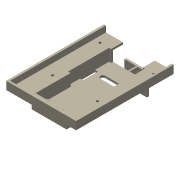
# Autodesk Inventor part: stat_plate
Saved by Autodesk Inventor 2022 (Build 260148000, 148)
## iProperties
Shininess: 64.0
Length Units: 11272
Angle Units: 11279
Time Units: 11290
Mass Units: 11286
Length Display Precision: 3
Angle Display Precision: 2
Created: 2002-04-25
Part Number: stat_plate
Document SubType Name: Modeling
Designer: Administrator
Density: 1 g/cm^3
Material: Generic
Appearance: Light Beige
Density: 0.0
Volumn: 0.0
Area: 0.0
PropertySet Name: Model Information
Control State: 0
Master: False
Checked Out: False
Author: Administrator
Autodesk Inventor part; units mm, degrees
ref_plane "YZ Plane" through (0, 0, 0) normal (1, 0, 0) x (0, 1, 0)
ref_plane "XZ Plane" through (0, 0, 0) normal (0, 1, 0) x (-1, 0, 0)
sketch "Sketch1" plane through (0, 0, 0) normal (0, 0, 1) x (1, 0, 0)
  line L0 (-52.4488, 14.7313) -> (-52.4488, 4.5713)
  line L1 (-52.4488, 4.5713) -> (36.4512, 4.5713)
  line L2 (36.4512, 4.5713) -> (36.4512, 14.7313)
  line L3 (36.4512, 14.7313) -> (-52.4488, 14.7313)
  dimension "d0" = 10.16
  dimension "d13" = 88.9
  constraints: 8 end point, 2 perpendicular, 1 horizontal, 1 parallel, 1 vertical
  measures "d0" distance of L0.start L0.end
  measures "d13" distance of L0.end L1.end
extrude "Extrusion1" add sketch "Sketch1" along normal blind 121.92
sketch "Sketch2" plane through (0, 0, 121.92) normal (0, 0, 1) x (1, 0, 0)
  line L0 (-52.4488, 14.7313) -> (-49.9088, 14.7313) projected
  line L1 (-52.4488, 4.5713) -> (-52.4488, 14.7313) projected
  line L2 (36.4512, 4.5713) -> (-52.4488, 4.5713) projected
  line L3 (36.4512, 14.7313) -> (36.4512, 4.5713) projected
  line L4 (33.9112, 14.7313) -> (36.4512, 14.7313) projected
  line L5 (33.9112, 7.1113) -> (33.9112, 14.7313) projected
  line L6 (-49.9088, 7.1113) -> (33.9112, 7.1113) projected
  line L7 (-49.9088, 14.7313) -> (-49.9088, 7.1113) projected
  line L8 (-52.4488, 4.5713) -> (36.4512, 4.5713)
  line L9 (36.4512, 4.5713) -> (36.4512, 14.7313)
  line L10 (36.4512, 14.7313) -> (-52.4488, 14.7313)
  line L11 (-52.4488, 14.7313) -> (-52.4488, 4.5713)
  constraints: 8 end point, 2 parallel, 1 horizontal, 1 perpendicular
extrude "Extrusion2" add sketch "Sketch2" along normal blind 2.54
sketch "Sketch3" plane through (-52.4488, 4.5713, 0) normal (0, -1, 0) x (1, 0, 0)
  line L0 (0, 0) -> (0, 124.46) projected
  line L1 (0, 0) -> (88.9, 0) projected
  line L2 (88.9, 0) -> (88.9, 124.46) projected
  line L3 (19.05, 69.85) -> (19.05, 12.7)
  line L4 (19.05, 12.7) -> (69.85, 12.7)
  line L5 (69.85, 12.7) -> (69.85, 69.85)
  circle A0 centre (44.45, 41.6186) radius 25.4 construction
  circle A1 centre (44.45, 41.6186) radius 44.45 construction
  line L6 (88.9, 124.46) -> (0, 124.46) projected
  line L7 (69.85, 69.85) -> (66.675, 69.85)
  line L8 (66.675, 69.85) -> (66.675, 114.3)
  line L9 (66.675, 114.3) -> (22.225, 114.3)
  line L10 (22.225, 114.3) -> (22.225, 69.85)
  line L11 (22.225, 69.85) -> (19.05, 69.85)
  circle A2 centre (44.45, 103.9228) radius 22.225 construction
  dimension "d8" = 57.15
  dimension "d9" = 12.7
  dimension "d62" = 44.45
  dimension "d63" = 101.6
  dimension "d64" = 50.8
  constraints: 16 end point, 6 tangent, 5 parallel, 3 centre point, 1 coincident, 1 collinear, 1 perpendicular, 1 vertical alignment
  measures "d8" distance of L4.end L5.end
  measures "d9" distance between parallel lines of L1 L4
  measures "d62" distance of L8.end L9.end
  measures "d63" distance between parallel lines of L4 L9
  measures "d64" distance of L3.end L4.end
extrude "Extrusion3" add sketch "Sketch3" along normal blind 15.24 contours L11 L10 L9 L8 L7 L5 L4 L3
shell "Shell1" thickness 2.54 removed faces 2 at (6.8179, 14.7313, 41.4867) at (6.8179, 7.9579, 0)
sketch "Sketch5" plane through (-52.4488, 4.5713, 0) normal (0, -1, 0) x (1, 0, 0)
  line L0 (0, 0) -> (88.9, 0) projected
  line L1 (47.2599, 0) -> (24.5184, 0)
  line L2 (0, 0) -> (0, 124.46) projected
  line L3 (88.9, 0) -> (88.9, 124.46) projected
  circle A0 centre (44.45, 5.5227) radius 20.32 construction
  circle A1 centre (44.45, 5.5227) radius 44.45 construction
  line L4 (24.13, 7.6275) -> (64.77, 7.6275)
  line L5 (64.77, 7.6275) -> (64.77, 0)
  line L6 (64.77, 0) -> (24.13, 0)
  line L7 (24.13, 0) -> (24.13, 7.6275)
  point P0 (13.97, 7.62)
  dimension "d35" = 40.64
  constraints: 10 end point, 4 tangent, 2 centre point, 2 collinear, 2 parallel, 1 concentric, 1 horizontal, 1 perpendicular, 1 point on line
  measures "d35" distance of L5.end L6.end
extrude "Extrusion5" cut sketch "Sketch5" against normal up to surface (2.54 mm away)
sketch "Sketch6" plane through (-52.4488, -10.6687, 0) normal (0, -1, 0) x (1, 0, 0)
  line L0 (69.85, 69.85) -> (69.85, 12.7) projected
  line L1 (19.05, 12.7) -> (69.85, 12.7)
  line L2 (69.85, 12.7) -> (69.85, 15.24)
  line L3 (69.85, 15.24) -> (19.05, 15.24)
  line L4 (19.05, 15.24) -> (19.05, 12.7)
  dimension "d19" = 2.54
  constraints: 8 end point, 2 parallel, 1 horizontal, 1 perpendicular, 1 point on line
  measures "d19" distance of L3.end L1.start
extrude "Extrusion6" add sketch "Sketch6" along normal blind 12.7
ref_plane "Work Plane1" through (17.4012, 4.5713, 2.54) normal (0, 0, -1) x (-1, 0, 0)
sketch "Sketch7" plane through (17.4012, 4.5713, 2.54) normal (0, 0, -1) x (-1, 0, 0)
  line L0 (9.525, -11.43) -> (41.275, -11.43)
  line L1 (41.275, -11.43) -> (41.275, -25.4)
  line L2 (41.275, -25.4) -> (9.525, -25.4)
  line L3 (9.525, -25.4) -> (9.525, -11.43)
  circle A0 centre (25.4, -26.6329) radius 15.875 construction
  circle A1 centre (25.4, -26.6329) radius 25.4 construction
  line L4 (0, 0) -> (0, -27.94) projected
  line L5 (50.8, 0) -> (50.8, -27.94) projected
  point P0 (-63.5, 0)
  dimension "flatlength" = 31.75
  dimension "d24" = 13.97
  dimension "d25" = 2.54
  constraints: 8 end point, 3 tangent, 2 centre point, 2 parallel, 1 coincident, 1 horizontal, 1 perpendicular, 2 other
  measures "flatlength" distance of L1.end L2.end
  measures "d24" distance of L2.end L0.start
  measures "d25" vertical distance of point (0, -27.94) L2.end
extrude "Extrusion7" add sketch "Sketch7" along normal blind 2.54
sketch "Sketch8" plane through (7.8762, -20.8287, 2.54) normal (1, 0, 0) x (0, 0, -1)
  line L0 (2.54, 0) -> (2.54, 13.97) projected
  line L1 (2.54, 0) -> (-12.7, 0)
  line L2 (-12.7, 0) -> (-12.7, -2.54)
  line L3 (-12.7, -2.54) -> (2.54, -2.54)
  line L4 (2.54, -2.54) -> (2.54, 0)
  line L5 (-12.7, 10.16) -> (-12.7, -2.54) projected
  line L6 (-12.7, -2.54) -> (-10.16, -2.54) projected
  dimension "d28" = 2.54
  constraints: 8 end point, 2 collinear, 2 parallel, 1 horizontal, 1 perpendicular, 1 point on line
  measures "d28" distance of L3.end L1.start
extrude "Extrusion8" add sketch "Sketch8" against normal blind 2.032
pattern_linear "Rectangular Pattern1" count 3 spacing 14.859 along (-1, 0, 0) of "Extrusion8"
sketch "Sketch9" plane through (0, 0, 0) normal (0, 0, -1) x (-1, 0, 0)
  line L0 (28.3188, 7.1113) -> (-12.3212, 7.1113)
  line L1 (-12.3212, 7.1113) -> (-12.3212, -8.1287)
  line L2 (-12.3212, -8.1287) -> (28.3188, -8.1287)
  line L3 (28.3188, -8.1287) -> (28.3188, 7.1113)
  line L4 (-12.3212, 4.5713) -> (-12.3212, 7.1113) projected
  line L5 (33.3988, -10.6687) -> (-17.4012, -10.6687) projected
  dimension "d37" = 2.54
  constraints: 8 end point, 2 parallel, 1 collinear, 1 horizontal, 1 perpendicular
  measures "d37" distance between parallel lines of L5 L2
extrude "Extrusion9" cut sketch "Sketch9" against normal up to surface (15.24 mm away)
sketch "Sketch10" plane through (-52.4488, -10.6687, 0) normal (0, -1, 0) x (1, 0, 0)
  line L0 (69.85, 69.85) -> (69.85, 15.24) projected
  line L1 (19.05, 15.24) -> (19.05, 69.85) projected
  line L2 (21.59, 33.02) -> (25.4, 33.02)
  line L3 (25.4, 33.02) -> (25.4, 52.07)
  line L4 (25.4, 52.07) -> (21.59, 52.07)
  line L5 (21.59, 52.07) -> (21.59, 33.02)
  line L6 (34.925, 33.02) -> (53.975, 33.02)
  arc A0 (53.975, 33.02) -> (53.975, 39.37) centre (53.975, 36.195) ccw
  line L7 (53.975, 39.37) -> (34.925, 39.37)
  arc A1 (34.925, 39.37) -> (34.925, 33.02) centre (34.925, 36.195) ccw
  line L8 (63.5, 33.02) -> (67.31, 33.02)
  line L9 (67.31, 33.02) -> (67.31, 52.07)
  line L10 (67.31, 52.07) -> (63.5, 52.07)
  line L11 (63.5, 52.07) -> (63.5, 33.02)
  circle A2 centre (44.45, 44.2562) radius 25.4 construction
  circle A3 centre (44.45, 44.2562) radius 19.05 construction
  line L12 (21.59, 15.24) -> (21.59, 67.31) projected
  circle A4 centre (44.45, 44.2562) radius 9.3033 construction
  point P0 (69.85, 12.7)
  point P1 (15.24, 67.31)
  dimension "d40" = 19.05
  dimension "d41" = 20.32
  dimension "d42" = 3.175
  dimension "d43" = 19.05
  dimension "d44" = 3.81
  dimension "d45" = 38.1
  constraints: 20 end point, 10 tangent, 5 centre point, 5 parallel, 4 collinear, 4 point on circle, 3 perpendicular, 2 coincident, 2 horizontal, 1 other
  measures "d40" distance of L8.end L9.end
  measures "d41" distance from line of point (69.85, 12.7) L8
  measures "d42" radius of A0
  measures "d43" distance of L6.start L6.end
  measures "d44" distance of L8.start L8.end
  measures "d45" distance between parallel lines of L11 L3
extrude "Extrusion10" cut sketch "Sketch10" against normal up to surface (2.54 mm away)
sketch "Sketch11" plane through (-52.4488, 4.5713, 124.46) normal (0, -1, 0) x (1, 0, 0)
  line L0 (0, -124.46) -> (0, 0) projected
  line L1 (0, -124.46) -> (24.13, -124.46) projected
  line L2 (19.05, -111.76) -> (19.05, -44.45) projected
  line L3 (73.025, -43.18) -> (15.875, -43.18)
  line L4 (15.875, -43.18) -> (10.16, -109.22)
  line L5 (10.16, -109.22) -> (78.74, -109.22)
  line L6 (78.74, -109.22) -> (73.025, -43.18)
  circle A0 centre (44.45, -43.18) radius 28.575 construction
  circle A1 centre (44.45, -83.7019) radius 44.45 construction
  circle A2 centre (44.45, -83.7019) radius 31.9622 construction
  line L7 (86.36, -124.46) -> (86.36, -2.54) projected
  line L8 (88.9, -124.46) -> (88.9, 0) projected
  point P0 (12.7, -44.45)
  dimension "d48" = 68.58
  dimension "d49" = 57.15
  dimension "d50" = 15.24
  dimension "d51" = 66.04
  constraints: 8 end point, 4 tangent, 2 centre point, 1 coincident, 1 horizontal, 1 horizontal alignment, 1 midpoint, 1 parallel, 1 vertical alignment, 3 other
  measures "d48" distance of L4.end L5.end
  measures "d49" distance of L3.start L3.end
  measures "d50" distance between parallel lines of L1 L5
  measures "d51" vertical distance of L3.end L4.end
hole "Hole1" at (-36.5738, 4.5713, 81.28) at (20.5762, 4.5713, 81.28) at (-42.2888, 4.5713, 15.24) at (26.2912, 4.5713, 15.24) direction (0, 1, 0) diameter 3.175 end through all
sketch "Sketch12" plane through (-6.9828, -20.8287, 12.7) normal (0, 1, 0) x (1, 0, 0)
  line L0 (0, 0) -> (-2.032, 0) projected
  line L1 (0, 10.16) -> (0, 0) projected
  line L2 (-2.032, 10.16) -> (0, 10.16) projected
  line L3 (-2.032, 10.16) -> (-2.032, 0) projected
extrude "Extrusion11" add sketch "Sketch12" along normal up to surface (12.7 mm away)
sketch "Sketch13" plane through (-27.6838, -8.1287, 111.76) normal (0, 1, 0) x (1, 0, 0)
  arc A0 (29.21, 72.39) -> (29.21, 78.74) centre (29.21, 75.565) ccw projected
  arc A1 (10.16, 78.74) -> (10.16, 72.39) centre (10.16, 75.565) ccw projected
  circle A2 centre (10.16, 5.715) radius 1.27
  circle A3 centre (29.21, 5.715) radius 1.27
  line L0 (-24.765, -12.7) -> (64.135, -12.7) projected
  dimension "d65" = 2.54
  dimension "d69" = 69.85
  constraints: 2 centre point, 2 vertical alignment, 1 equal radius, 1 horizontal alignment
  measures "d65" diameter of A2
  measures "d69" distance of A2.centre A1.centre
extrude "Extrusion12" add sketch "Sketch13" along normal blind 10.16
equation "\"d33\" = -0.5 * ribthick + 0.5 * flatlength"
equation "\"ribthick\" = 2.032"
body "Solid1"
